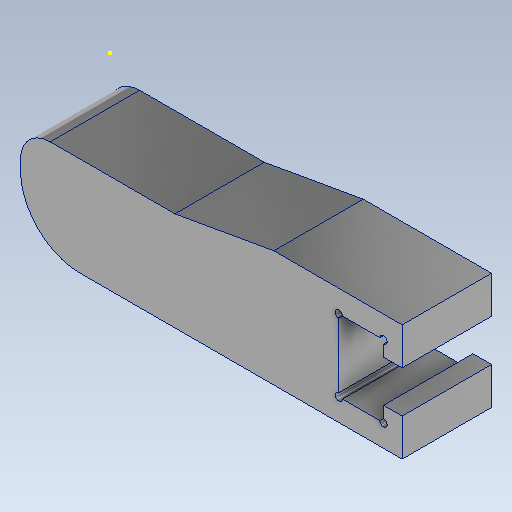
# Autodesk Inventor part: Finray_9_Kerbe_10deg_anschluss_erweitert_9_75 Nut
Saved by Autodesk Inventor 2025.2 (Build 292293000, 293)
## iProperties
Created: 2022-02-28
Part Number: Finray_9_Kerbe_10deg_anschluss_erweitert_9_75 Nut
Material: Generic
Document SubType Name: Modeling
Designer: richa
Density: 1 g/cm^3
Appearance: Aluminum - Flat
Author: richa
## iProperties of the stored document Maria_Greifer_Dreieck2_3D-Druck.ipt
Created: 2024-11-23
Part Number: Maria_Greifer_Dreieck2_3D-Druck
Material: Generisch
Document SubType Name: Modeling
Designer: maria
Density: 1 g/cm^3
Appearance: Vorgabe
Author: maria
Autodesk Inventor part; units mm, degrees
ref_plane "YZ Plane" through (0, 0, 0) normal (1, 0, 0) x (0, 1, 0)
ref_plane "XZ Plane" through (0, 0, 0) normal (0, 1, 0) x (-1, 0, 0)
ref_plane "XY Plane" through (0, 0, 0) normal (0, 0, 1) x (1, 0, 0)
sketch "Sketch5" plane through (0, 0, 0) normal (0, 0, 1) x (1, 0, 0)
  line L0 (51.2279, -15.6) -> (51.2279, -10.6)
  line L1 (51.2279, -10.6) -> (48.7279, -10.6)
  line L2 (48.7279, -10.6) -> (48.7279, -12.625)
  line L3 (42.7279, -12.625) -> (42.7279, -2.975)
  line L4 (48.7279, -2.975) -> (48.7279, -5)
  line L5 (48.7279, -5) -> (51.2279, -5)
  line L6 (51.2279, -5) -> (51.2279, 0)
  line L7 (42.7279, -2.975) -> (48.7279, -2.975)
  line L8 (42.7279, -12.625) -> (48.7279, -12.625)
  line L9 (51.2279, -15.6) -> (43.6357, -15.6)
  line L10 (39.8786, -15.6) -> (43.6357, -15.6)
  line L11 (0, -15.6) -> (39.8786, -15.6)
  line L12 (36.9909, 0) -> (51.2279, 0)
  line L13 (0, -15.6) -> (0, -5.4692)
  line L14 (36.9909, 0) -> (31.0226, 0)
  line L15 (34.0067, 0) -> (20.7329, -2.3405)
  line L16 (0, -5.4692) -> (0, -2.3405)
  line L17 (0, -2.3405) -> (20.7329, -2.3405)
  point P0 (0, 0)
  point P1 (44.1094, 0)
  dimension "d41" = 6
  dimension "d50" = 2.5
  dimension "d87" = 5.6
  dimension "d88" = 9.65
  dimension "d122" = 14.237
  dimension "d123" = 2.975
  dimension "d132" = 10
  constraints: 36 end point, 7 perpendicular, 5 collinear, 3 horizontal, 3 parallel, 3 vertical, 2 midpoint
  measures "d41" distance between parallel lines of L2 L3
  measures "d50" distance of L4.end L5.end
  measures "d87" distance from line of L0.end L5
  measures "d88" distance of L3.start L3.end
  measures "d122" distance of L12.start L6.end
  measures "d123" distance from line of point (44.109, 0) L7
  measures "d132" angle of L15 L12
extrude "Extrusion2" add sketch "Sketch5" along normal blind 12
sketch "Sketch11" plane through (0, 0, 12) normal (0, 0, 1) x (1, 0, 0)
  line L0 (42.7279, -2.975) -> (48.7279, -2.975) projected
  circle A0 centre (42.7279, -2.975) radius 0.5
  line L1 (42.7279, -12.625) -> (42.7279, -2.975) projected
  circle A1 centre (42.7279, -12.625) radius 0.5
  line L2 (48.7279, -12.625) -> (42.7279, -12.625) projected
  circle A2 centre (48.7279, -12.625) radius 0.5
  line L3 (48.7279, -2.975) -> (48.7279, -5) projected
  circle A3 centre (48.7279, -2.975) radius 0.5
  point P0 (0, 0)
  dimension "d99" = 1
  dimension "d100" = 1
  dimension "d101" = 1
  dimension "d102" = 1
  constraints: 4 centre point, 1 coincident
  measures "d99" diameter of A0
  measures "d100" diameter of A1
  measures "d101" diameter of A2
  measures "d102" diameter of A3
extrude "Extrusion7" cut sketch "Sketch11" against normal through all
fillet "Rundung4" radius 8 1 edges at (0, -15.6, 6)
sketch "Skizze13" plane through (0, 0, 0) normal (-1, 0, 0) x (0, 0, 1)
  point P0 (0, 0)
fillet "Rundung7" radius 4 1 edges at (0, -2.3405, 6)
equation "\"l1\" = 8"
body "Solid2"
